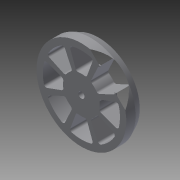
# Autodesk Inventor part: Colossus_7kW_Rotor
Saved by Autodesk Inventor 2014 (Build 180170000, 170)
## iProperties
Created: 2014-11-23
Part Number: Colossus_7kW_Rotor
Material: Générique
Document SubType Name: Modeling
Designer: Yann
Density: 1 g/cm^3
Appearance: Par défaut
Author: Yann
Autodesk Inventor part; units mm, degrees
ref_plane "YZ Plane" through (0, 0, 0) normal (1, 0, 0) x (0, 1, 0)
ref_plane "XZ Plane" through (0, 0, 0) normal (0, 1, 0) x (-1, 0, 0)
ref_plane "XY Plane" through (0, 0, 0) normal (0, 0, 1) x (1, 0, 0)
sketch "Esquisse1" plane through (0, 0, 0) normal (0, 1, 0) x (-1, 0, 0)
  arc A0 (26.7424, 50.7333) -> (-26.7424, 50.7333) centre (0, 0) ccw
  circle A1 centre (0, 0) radius 57.35
  line L0 (0, -80.29) -> (0, 80.29) construction
  line L1 (-80.29, 0) -> (80.29, 0) construction
  circle A2 centre (0, 0) radius 4
  line L2 (-7.3279, 25.1704) -> (-14.1513, 43.9173)
  line L3 (14.1513, 43.9173) -> (7.3279, 25.1704)
  arc A3 (12.0657, 47.8523) -> (-12.0657, 47.8523) centre (0, 0) ccw
  arc A4 (-12.0657, 47.8523) -> (-14.1513, 43.9173) centre (-11.3322, 44.9433) ccw
  arc A5 (14.1513, 43.9173) -> (12.0657, 47.8523) centre (11.3322, 44.9433) ccw
  circle A6 centre (0, 0) radius 16 construction
  circle A7 centre (0, 0) radius 57.35 construction
  arc A8 (4, 23.2399) -> (-4, 23.2399) centre (0, 0) ccw
  arc A9 (-7.3279, 25.1704) -> (-4, 23.2399) centre (-4.5089, 26.1964) ccw
  arc A10 (4, 23.2399) -> (7.3279, 25.1704) centre (4.5089, 26.1964) ccw
  line L4 (-22.9798, 12.6165) -> (-41.0607, 21.0478)
  line L5 (-21.0478, 41.0607) -> (-12.6165, 22.9798)
  arc A11 (-25.305, 42.3684) -> (-42.3684, 25.305) centre (0, 0) ccw
  arc A12 (-42.3684, 25.305) -> (-41.0607, 21.0478) centre (-39.7928, 23.7667) ccw
  arc A13 (-21.0478, 41.0607) -> (-25.305, 42.3684) centre (-23.7667, 39.7928) ccw
  arc A14 (-13.6047, 19.2615) -> (-19.2615, 13.6047) centre (0, 0) ccw
  arc A15 (-22.9798, 12.6165) -> (-19.2615, 13.6047) centre (-21.7119, 15.3354) ccw
  arc A16 (-13.6047, 19.2615) -> (-12.6165, 22.9798) centre (-15.3354, 21.7119) ccw
  line L6 (-25.1704, -7.3279) -> (-43.9173, -14.1513)
  line L7 (-43.9173, 14.1513) -> (-25.1704, 7.3279)
  arc A17 (-47.8523, 12.0657) -> (-47.8523, -12.0657) centre (0, 0) ccw
  arc A18 (-47.8523, -12.0657) -> (-43.9173, -14.1513) centre (-44.9433, -11.3322) ccw
  arc A19 (-43.9173, 14.1513) -> (-47.8523, 12.0657) centre (-44.9433, 11.3322) ccw
  arc A20 (-23.2399, 4) -> (-23.2399, -4) centre (0, 0) ccw
  arc A21 (-25.1704, -7.3279) -> (-23.2399, -4) centre (-26.1964, -4.5089) ccw
  arc A22 (-23.2399, 4) -> (-25.1704, 7.3279) centre (-26.1964, 4.5089) ccw
  line L8 (-12.6165, -22.9798) -> (-21.0478, -41.0607)
  line L9 (-41.0607, -21.0478) -> (-22.9798, -12.6165)
  arc A23 (-42.3684, -25.305) -> (-25.305, -42.3684) centre (0, 0) ccw
  arc A24 (-25.305, -42.3684) -> (-21.0478, -41.0607) centre (-23.7667, -39.7928) ccw
  arc A25 (-41.0607, -21.0478) -> (-42.3684, -25.305) centre (-39.7928, -23.7667) ccw
  arc A26 (-19.2615, -13.6047) -> (-13.6047, -19.2615) centre (0, 0) ccw
  arc A27 (-12.6165, -22.9798) -> (-13.6047, -19.2615) centre (-15.3354, -21.7119) ccw
  arc A28 (-19.2615, -13.6047) -> (-22.9798, -12.6165) centre (-21.7119, -15.3354) ccw
  line L10 (7.3279, -25.1704) -> (14.1513, -43.9173)
  line L11 (-14.1513, -43.9173) -> (-7.3279, -25.1704)
  arc A29 (-12.0657, -47.8523) -> (12.0657, -47.8523) centre (0, 0) ccw
  arc A30 (12.0657, -47.8523) -> (14.1513, -43.9173) centre (11.3322, -44.9433) ccw
  arc A31 (-14.1513, -43.9173) -> (-12.0657, -47.8523) centre (-11.3322, -44.9433) ccw
  arc A32 (-4, -23.2399) -> (4, -23.2399) centre (0, 0) ccw
  arc A33 (7.3279, -25.1704) -> (4, -23.2399) centre (4.5089, -26.1964) ccw
  arc A34 (-4, -23.2399) -> (-7.3279, -25.1704) centre (-4.5089, -26.1964) ccw
  line L12 (22.9798, -12.6165) -> (41.0607, -21.0478)
  line L13 (21.0478, -41.0607) -> (12.6165, -22.9798)
  arc A35 (25.305, -42.3684) -> (42.3684, -25.305) centre (0, 0) ccw
  arc A36 (42.3684, -25.305) -> (41.0607, -21.0478) centre (39.7928, -23.7667) ccw
  arc A37 (21.0478, -41.0607) -> (25.305, -42.3684) centre (23.7667, -39.7928) ccw
  arc A38 (13.6047, -19.2615) -> (19.2615, -13.6047) centre (0, 0) ccw
  arc A39 (22.9798, -12.6165) -> (19.2615, -13.6047) centre (21.7119, -15.3354) ccw
  arc A40 (13.6047, -19.2615) -> (12.6165, -22.9798) centre (15.3354, -21.7119) ccw
  line L14 (25.1704, 7.3279) -> (43.9173, 14.1513)
  line L15 (43.9173, -14.1513) -> (25.1704, -7.3279)
  arc A41 (47.8523, -12.0657) -> (47.8523, 12.0657) centre (0, 0) ccw
  arc A42 (47.8523, 12.0657) -> (43.9173, 14.1513) centre (44.9433, 11.3322) ccw
  arc A43 (43.9173, -14.1513) -> (47.8523, -12.0657) centre (44.9433, -11.3322) ccw
  arc A44 (23.2399, -4) -> (23.2399, 4) centre (0, 0) ccw
  arc A45 (25.1704, 7.3279) -> (23.2399, 4) centre (26.1964, 4.5089) ccw
  arc A46 (23.2399, -4) -> (25.1704, -7.3279) centre (26.1964, -4.5089) ccw
  line L16 (12.6165, 22.9798) -> (21.0478, 41.0607)
  line L17 (41.0607, 21.0478) -> (22.9798, 12.6165)
  arc A47 (42.3684, 25.305) -> (25.305, 42.3684) centre (0, 0) ccw
  arc A48 (25.305, 42.3684) -> (21.0478, 41.0607) centre (23.7667, 39.7928) ccw
  arc A49 (41.0607, 21.0478) -> (42.3684, 25.305) centre (39.7928, 23.7667) ccw
  arc A50 (19.2615, 13.6047) -> (13.6047, 19.2615) centre (0, 0) ccw
  arc A51 (12.6165, 22.9798) -> (13.6047, 19.2615) centre (15.3354, 21.7119) ccw
  arc A52 (19.2615, 13.6047) -> (22.9798, 12.6165) centre (21.7119, 15.3354) ccw
  point P0 (0, 0)
  point P1 (-15.2495, 46.9348)
  point P2 (15.2495, 46.9348)
  point P3 (6.425, 22.6895)
  point P4 (-6.425, 22.6895)
  point P5 (-43.971, 22.4048)
  point P6 (-22.4048, 43.971)
  point P7 (-11.5007, 20.587)
  point P8 (-20.587, 11.5007)
  point P9 (-46.9348, -15.2495)
  point P10 (-46.9348, 15.2495)
  point P11 (-22.6895, 6.425)
  point P12 (-22.6895, -6.425)
  point P13 (-22.4048, -43.971)
  point P14 (-43.971, -22.4048)
  point P15 (-20.587, -11.5007)
  point P16 (-11.5007, -20.587)
  point P17 (15.2495, -46.9348)
  point P18 (-15.2495, -46.9348)
  point P19 (-6.425, -22.6895)
  point P20 (6.425, -22.6895)
  point P21 (43.971, -22.4048)
  point P22 (22.4048, -43.971)
  point P23 (11.5007, -20.587)
  point P24 (20.587, -11.5007)
  point P25 (46.9348, 15.2495)
  point P26 (46.9348, -15.2495)
  point P27 (22.6895, -6.425)
  point P28 (22.6895, 6.425)
  point P29 (22.4048, 43.971)
  point P30 (43.971, 22.4048)
  point P31 (20.587, 11.5007)
  point P32 (11.5007, 20.587)
  dimension "d0" = 8
  dimension "d2" = 3
  dimension "d3" = 8
  dimension "d5" = 40
  dimension "d15" = 23.5816
  dimension "d16" = 3
  dimension "d17" = 8
  dimension "d20" = 360
  constraints: 130 point on circle, 51 centre point, 32 end point, 32 point on line, 9 tangent, 5 coincident, 3 equal radius, 1 symmetric about line, 210 other
  measures "d0" diameter of A2
  measures "d2" radius of A4
  measures "d3" radial gap between concentric circles of A3 A1
  measures "d5" angle of L3 L2
  measures "d15" radius of A8
  measures "d16" radius of A9
  measures "d17" distance of A8.start A8.end
extrude "Extrusion1" add sketch "Esquisse1" against normal blind 22
chamfer "Chanfrein1" distance 10 angle 25 1 edges at (57.35, 0, 0) measured on face at (57.35, -0.5, 0)
